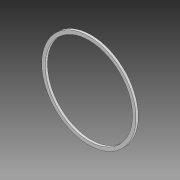
# Autodesk Inventor part: HD_GapFillSpacer
Saved by Autodesk Inventor 2020 (Build 240168000, 168)
## iProperties
Created: 2021-04-18
Part Number: HD_GapFillSpacer
Material: Generic
Document SubType Name: Modeling
Designer: DDeGo
Density: 1 g/cm^3
Appearance: Default
Author: DDeGo
Autodesk Inventor part; units mm, degrees
ref_plane "YZ Plane" through (0, 0, 0) normal (1, 0, 0) x (0, 1, 0)
ref_plane "XZ Plane" through (0, 0, 0) normal (0, 1, 0) x (-1, 0, 0)
ref_plane "XY Plane" through (0, 0, 0) normal (0, 0, 1) x (1, 0, 0)
sketch "Sketch2" plane through (0, 0, 0) normal (0, 0, 1) x (1, 0, 0)
  circle A0 centre (0, 0) radius 37.75
  circle A1 centre (0, 0) radius 40.75
  dimension "d7" = 75.5
  dimension "d8" = 3
  constraints: 2 centre point, 2 coincident
  measures "d7" diameter of A0
  measures "d8" radial gap between concentric circles of A1 A0
extrude "Extrusion1" add sketch "Sketch2" along normal blind 2
body "Solid2"
